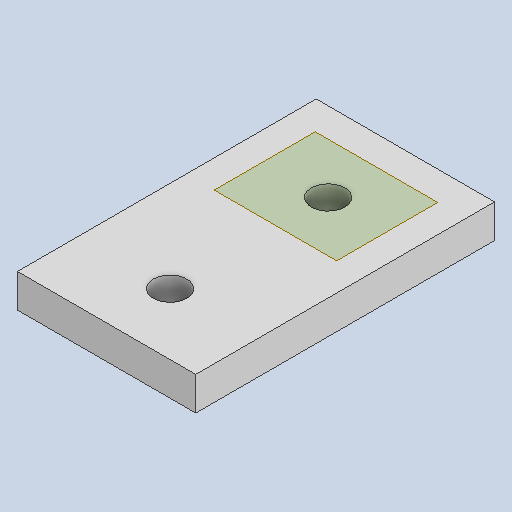
# Autodesk Inventor part: деталь закрывает
Saved by Autodesk Inventor 2024.2 (Build 282272000, 272)
## iProperties
Created: 2026-02-05
Part Number: деталь закрывает
Material: Типовые
Document SubType Name: Modeling
Designer: katya_notebook
Density: 1 g/cm^3
Appearance: По умолчанию
Author: katya_notebook
Autodesk Inventor part; units mm, degrees
ref_plane "YZ Plane" through (0, 0, 0) normal (1, 0, 0) x (0, 1, 0)
ref_plane "XZ Plane" through (0, 0, 0) normal (0, 1, 0) x (-1, 0, 0)
ref_plane "XY Plane" through (0, 0, 0) normal (0, 0, 1) x (1, 0, 0)
ref_plane "РабПлоскость1" through (191.4757, 214.7821, 31.0958) normal (0, -1, 0) x (1, 0, 0)
sketch "Эскиз1" plane through (191.4757, 214.7821, 31.0958) normal (0, -1, 0) x (1, 0, 0)
  circle A0 centre (0.1884, -6.27) radius 1.5 projected
  arc A1 (-4.9877, -8.385) -> (-2.9877, -10.385) centre (-2.9877, -8.385) ccw projected
  line L0 (4.9877, -10.385) -> (-2.9877, -10.385) projected
  line L1 (4.9877, -2.155) -> (4.9877, -10.385) projected
  line L2 (-4.9877, -2.155) -> (4.9877, -2.155) projected
  line L3 (-4.9877, -8.385) -> (-4.9877, -2.155) projected
  circle A2 centre (0.1884, 7.885) radius 1.5 projected
  line L4 (-4.9877, 5.385) -> (-4.9877, 10.385) projected
  line L5 (4.9877, 5.385) -> (-4.9877, 5.385) projected
  line L6 (4.9877, 10.385) -> (4.9877, 5.385) projected
  line L7 (-4.9877, 10.385) -> (4.9877, 10.385) projected
  line L8 (7.9877, -13.385) -> (-7.9877, -13.385)
  line L9 (-7.9877, -13.385) -> (-7.9877, 13.385)
  line L10 (-7.9877, 13.385) -> (7.9877, 13.385)
  line L11 (7.9877, 13.385) -> (7.9877, -13.385)
  point P0 (-191.4757, -31.0958)
  dimension "d0" = 3
  dimension "d1" = 3
  dimension "d2" = 3
  dimension "d3" = 3
  constraints: 8 end point, 2 parallel, 1 horizontal, 1 perpendicular
  measures "d0" distance between parallel lines of L7 L10
  measures "d1" distance between parallel lines of L8 L0
  measures "d2" distance between parallel lines of L11 L6
  measures "d3" distance between parallel lines of L9 L4
extrude "Выдавливание1" add sketch "Эскиз1" along normal blind 3 contours L3 L2 L1 L0 A1 | L4 L7 L6 L5 | L8 L9 L10 L11
